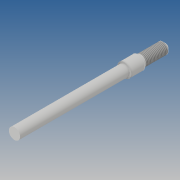
# Autodesk Inventor part: cartridge_locker_piston_axe
Saved by Autodesk Inventor 2019 (Build 230136000, 136)
## iProperties
Created: 2019-03-17
Part Number: cartridge_locker_piston_axe
Material: Générique
Document SubType Name: Modeling
Designer: Theo
Density: 1 g/cm^3
Appearance: Par défaut
Author: Theo
Autodesk Inventor part; units mm, degrees
ref_plane "YZ Plane" through (0, 0, 0) normal (1, 0, 0) x (0, 1, 0)
ref_plane "XZ Plane" through (0, 0, 0) normal (0, 1, 0) x (-1, 0, 0)
ref_plane "XY Plane" through (0, 0, 0) normal (0, 0, 1) x (1, 0, 0)
sketch "Esquisse2" plane through (0, 0, 0) normal (1, 0, 0) x (0, 1, 0)
  line L0 (0, 0) -> (0, 55)
  line L1 (0, 0) -> (2, 0)
  line L2 (2, 0) -> (2, 10)
  line L3 (2, 10) -> (2.5, 10)
  line L4 (2.5, 10) -> (2.5, 15)
  line L5 (2.5, 15) -> (2, 15)
  line L6 (2, 15) -> (2, 55)
  line L7 (2, 55) -> (0, 55)
  dimension "d3" = 10
  dimension "d4" = 0.5
  dimension "d5" = 2
  dimension "d6" = 5
  dimension "d20" = 40
  constraints: 16 end point, 4 horizontal, 4 vertical, 1 collinear
  measures "d3" distance of L1.end L2.end
  measures "d4" distance of L2.end L3.end
  measures "d5" distance between parallel lines of L6 L0
  measures "d6" distance between parallel lines of L5 L3
  measures "d20" distance between parallel lines of L7 L5
revolve "Révolution1" add sketch "Esquisse2" angle 360 about axis through (0, 0, 0) along (0, 0, 1)
thread "Filetage1" size "M4x0.5" class "6g" standard "ANSI Metric M Profile" length 9
chamfer "Chanfrein1" distance 1 angle 45 1 edges at (0, -2, 0)
